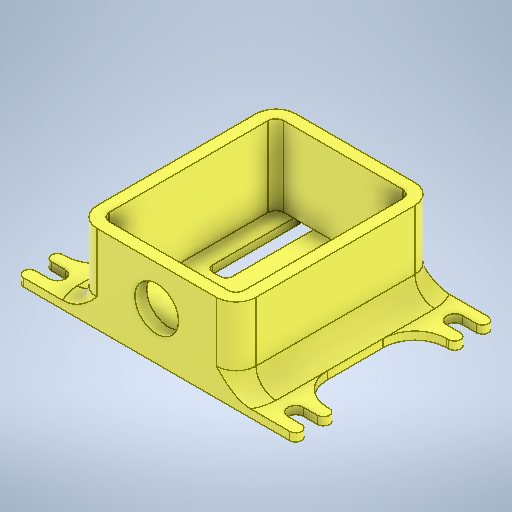
# Autodesk Inventor part: RT_ELE_PR_016_ESTOP_Enclosure
Saved by Autodesk Inventor 2025.3 (Build 293356000, 356)
## iProperties
Created: 2026-06-07
Part Number: RT_ELE_PR_016_ESTOP_Enclosure
Material: ABS Plastic
Document SubType Name: Modeling
Designer: louis
Density: 1.06 g/cm^3
Appearance: Smooth - Yellow
Author: louis
Autodesk Inventor part; units mm, degrees
ref_plane "YZ Plane" through (0, 0, 0) normal (1, 0, 0) x (0, 1, 0)
ref_plane "XZ Plane" through (0, 0, 0) normal (0, 1, 0) x (-1, 0, 0)
ref_plane "XY Plane" through (0, 0, 0) normal (0, 0, 1) x (1, 0, 0)
sketch "Sketch1" plane through (0, 0, 0) normal (0, 0, 1) x (1, 0, 0)
  line L0 (-50, -50) -> (50, -50)
  line L1 (50, -50) -> (50, 50)
  line L2 (50, 50) -> (-50, 50)
  line L3 (-50, 50) -> (-50, -50)
  line L4 (-50, -50) -> (50, 50) construction
  line L5 (50, -50) -> (-50, 50) construction
  line L6 (-20, 50) -> (20, 50)
  line L7 (20, 50) -> (20, -50)
  line L8 (20, -50) -> (-20, -50)
  line L9 (-20, -50) -> (-20, 50)
  line L10 (0, 0) -> (0, 50) construction
  line L11 (-25, 50) -> (-15, 50) construction
  line L12 (-15, 50) -> (-15, 0)
  line L13 (-15, 0) -> (-25, 0)
  line L14 (-25, 0) -> (-25, 50)
  line L15 (-50, 50) -> (-70, 50)
  line L16 (-70, 50) -> (-70, 30)
  line L17 (-70, 30) -> (-50, 30)
  line L18 (-50, 30) -> (-50, 50) construction
  circle A0 centre (-60, 40) radius 4
  line L19 (-60, 40) -> (-60, 50) construction
  line L20 (-60, 40) -> (-60, 30) construction
  line L21 (-60, 44) -> (-70, 44)
  line L22 (-60, 36) -> (-70, 36)
  line L23 (-15, 0) -> (0, 0) construction
  line L24 (-50, -50) -> (-70, -50)
  line L25 (-70, -50) -> (-70, -30)
  line L26 (-70, -30) -> (-50, -30)
  line L27 (-50, -30) -> (-50, -50) construction
  circle A1 centre (-60, -40) radius 4
  line L28 (-60, -40) -> (-60, -50) construction
  line L29 (-60, -40) -> (-60, -30) construction
  line L30 (-60, -44) -> (-70, -44)
  line L31 (-60, -36) -> (-70, -36)
  line L32 (50, 50) -> (50, -50)
  line L33 (50, 50) -> (70, 50)
  line L34 (70, 50) -> (70, 30)
  line L35 (70, 30) -> (50, 30)
  line L36 (50, 30) -> (50, 50) construction
  circle A2 centre (60, 40) radius 4
  line L37 (60, 40) -> (60, 50) construction
  line L38 (60, 40) -> (60, 30) construction
  line L39 (60, 44) -> (70, 44)
  line L40 (60, 36) -> (70, 36)
  line L41 (50, -30) -> (50, -50) construction
  line L42 (60, -40) -> (60, -30) construction
  line L43 (70, -30) -> (50, -30)
  circle A3 centre (60, -40) radius 4
  line L44 (60, -36) -> (70, -36)
  line L45 (60, -40) -> (60, -50) construction
  line L46 (50, -50) -> (70, -50)
  line L47 (60, -44) -> (70, -44)
  line L48 (70, -50) -> (70, -30)
  point P0 (50, -30)
  point P1 (50, 30)
  point P2 (-15, 50)
  dimension "d0" = 100
  dimension "d1" = 100
  dimension "d2" = 40
  dimension "d3" = 10
  dimension "d4" = 20
  dimension "d5" = 20
  dimension "d6" = 8
  dimension "d7" = 10
  constraints: 98 end point, 30 symmetric about line, 19 point on line, 11 midpoint, 8 parallel, 8 perpendicular, 8 point on circle, 5 horizontal, 4 centre point, 2 tangent, 1 collinear, 1 vertical, 5 other
  measures "d0" distance of L2.end L1.end
  measures "d1" distance of L1.end L0.end
  measures "d2" distance between parallel lines of L9 L7
  measures "d3" distance of L12.end L13.end
  measures "d4" distance of L17.end L16.end
  measures "d5" distance of L16.end L15.end
  measures "d6" diameter of A0
  measures "d7" distance between parallel lines of L18 L19
extrude "Extrusion1" add sketch "Sketch1" along normal blind 4 contours L3 L2 L14 L13 L9 L0 | L24 L25 L30 A1 L31 L26 L3 | L9 L13 L12 L2 L7 L0 | L7 L2 L1 L0 | L17 L16 L22 A0 L21 L15 L3 | L1 L43 L48 L44 A3 L47 L46 | L33 L34 L39 A2 L40 L35 L1
fillet "Fillet1" radius 3 20 edges at (-70, -30, 2) (-70, -44, 2) (-70, -36, 2) (-70, -50, 2) (-70, 30, 2) (-70, 36, 2) (-70, 50, 2) (-70, 44, 2) (-25, 50, 2) (-15, 50, 2) (70, 50, 2) (70, 36, 2) (70, 30, 2) (70, -30, 2) (70, -44, 2) (70, -36, 2) (70, -50, 2) (70, 44, 2) (-25, 0, 2) (-15, 0, 2)
fillet "Fillet2" radius 16 4 edges at (-50, 30, 2) (-50, -30, 2) (50, -30, 2) (50, 30, 2)
sketch "Sketch2" plane through (0, 0, 4) normal (0, 0, 1) x (1, 0, 0)
  line L0 (-30, -50) -> (30, -50)
  line L1 (40, -40) -> (40, 40)
  line L2 (30, 50) -> (-30, 50)
  line L3 (-40, 40) -> (-40, -40)
  line L4 (-40, -50) -> (40, 50) construction
  line L5 (40, -50) -> (-40, 50) construction
  arc A0 (-30, 50) -> (-40, 40) centre (-30, 40) ccw
  arc A1 (40, 40) -> (30, 50) centre (30, 40) ccw
  arc A2 (30, -50) -> (40, -40) centre (30, -40) ccw
  arc A3 (-40, -40) -> (-30, -50) centre (-30, -40) ccw
  line L6 (-34, 40) -> (-34, -40)
  arc A4 (-34, -40) -> (-30, -44) centre (-30, -40) ccw
  line L7 (-30, -44) -> (30, -44)
  arc A5 (30, -44) -> (34, -40) centre (30, -40) ccw
  line L8 (34, -40) -> (34, 40)
  arc A6 (34, 40) -> (30, 44) centre (30, 40) ccw
  line L9 (30, 44) -> (-30, 44)
  arc A7 (-30, 44) -> (-34, 40) centre (-30, 40) ccw
  point P0 (0, 0)
  dimension "d13" = 80
  dimension "d14" = 100
  dimension "d15" = 10
  dimension "d16" = 10
  dimension "d17" = 6
  constraints: 20 end point, 16 point on circle, 8 centre point, 8 point on line, 8 tangent, 4 parallel, 2 equal radius, 2 midpoint, 2 perpendicular, 1 horizontal, 7 other
  measures "d13" distance of L5.end L4.end
  measures "d14" distance of L4.end L5.start
  measures "d15" radius of A0
  measures "d16" radius of A1
  measures "d17" radial gap between concentric circles of A0 A7
extrude "Extrusion2" add sketch "Sketch2" along normal blind 40
sketch "Sketch3" plane through (-67, -50, 0) normal (0, -1, 0) x (1, 0, 0)
  line L0 (37, 4) -> (37, 44) construction
  line L1 (97, 44) -> (101, 44) construction
  line L2 (37, 4) -> (97, 44) construction
  circle A0 centre (67, 24) radius 11
  point P0 (67, 0)
  dimension "d20" = 22
  constraints: 2 end point, 2 midpoint, 1 centre point
  measures "d20" diameter of A0
extrude "Extrusion3" cut sketch "Sketch3" against normal blind 40
fillet "Fillet3" radius 10 6 edges at (-40, 0, 4) (-37.0711, 47.0711, 4) (-37.0711, -47.0711, 4) (40, 0, 4) (37.0711, 47.0711, 4) (37.0711, -47.0711, 4)
equation "\"d15\" = d16"
body "Solid1"
